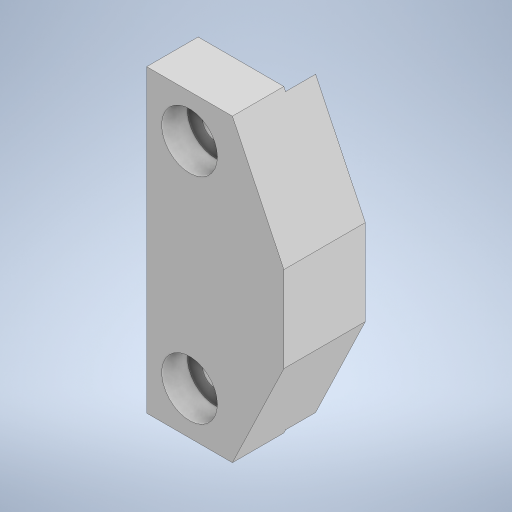
# Autodesk Inventor part: Clamp
Saved by Autodesk Inventor 2024 (Build 280153000, 153)
## iProperties
Created: 2024-09-24
Part Number: Clamp
Material: Generic
Document SubType Name: Modeling
Designer: Kemper Room 121
Density: 1 g/cm^3
Appearance: Default
Author: Kemper Room 121
Autodesk Inventor part; units mm, degrees
ref_plane "YZ Plane" through (0, 0, 0) normal (1, 0, 0) x (0, 1, 0)
ref_plane "XZ Plane" through (0, 0, 0) normal (0, 1, 0) x (-1, 0, 0)
ref_plane "XY Plane" through (0, 0, 0) normal (0, 0, 1) x (1, 0, 0)
sketch "Sketch1" plane through (0, 0, 0) normal (0, 0, 1) x (1, 0, 0)
  line L0 (0, 0) -> (0, 5)
  line L1 (0, 5) -> (0, 30)
  line L2 (0, 30) -> (0, 35)
  line L3 (0, 35) -> (10, 35)
  line L4 (10, 35) -> (10, 0)
  line L5 (10, 0) -> (0, 0)
  line L6 (0, 35) -> (5, 35)
  line L7 (5, 35) -> (5, 0)
  circle A0 centre (5, 30) radius 1.5
  circle A1 centre (5, 5) radius 1.5
  line L8 (5, 17.5) -> (10, 17.5)
  line L9 (10, 17.5) -> (16, 17.5)
  line L10 (16, 17.5) -> (16, 12.5)
  line L11 (16, 17.5) -> (16, 22.5)
  line L12 (16, 22.5) -> (10, 35)
  line L13 (16, 12.5) -> (10, 0)
  dimension "d0" = 5
  dimension "d1" = 25
  dimension "d2" = 5
  dimension "d3" = 10
  dimension "d4" = 5
  dimension "d5" = 3
  dimension "d6" = 3
  dimension "d7" = 6
  dimension "d8" = 5
  dimension "d9" = 5
  constraints: 28 end point, 4 midpoint, 4 point on line, 3 perpendicular, 3 vertical, 2 centre point, 1 horizontal
  measures "d0" distance of L0.start L0.end
  measures "d1" distance of L0.end L1.end
  measures "d2" distance of L1.end L2.end
  measures "d3" distance of L2.end L3.end
  measures "d4" distance of L2.end L6.end
  measures "d5" diameter of A0
  measures "d6" diameter of A1
  measures "d7" distance of L8.end L9.end
  measures "d8" distance of L9.end L10.end
  measures "d9" distance of L9.end L11.end
extrude "Extrusion1" add sketch "Sketch1" along normal blind 6 contours L0 L1 L2 L3 L7 A0 A1 L5 | L7 A1 L8 L4 L5 | L4 L9 L10 L13 | L8 L7 A0 L3 L4 | L4 L12 L11 L9
sketch "Sketch2" plane through (0, 0, 0) normal (0, 0, -1) x (-1, 0, 0)
  line L0 (0, 35) -> (0, 0) projected
  line L1 (-10, 35) -> (0, 35) projected
  line L2 (-16, 22.5) -> (-10, 35) projected
  line L3 (-16, 12.5) -> (-16, 22.5) projected
  line L4 (-10, 0) -> (-16, 12.5) projected
  line L5 (0, 0) -> (-10, 0) projected
  circle A0 centre (-5, 30) radius 1.5 projected
  circle A1 centre (-5, 5) radius 1.5 projected
  line L6 (-10, 0) -> (-16, 12.5) projected
  line L7 (-10, 35) -> (-10, 0)
  line L8 (-10, 0) -> (-16, 12.5)
  line L9 (-16, 12.5) -> (-16, 22.5)
  line L10 (-10, 35) -> (-16, 22.5)
  line L11 (-10.2, 34.5833) -> (-10.2, 0.4167)
  point P0 (-10.2, 0.4167)
  dimension "d54" = 0.2
  constraints: 10 end point, 2 parallel, 2 point on line, 1 collinear, 1 vertical
  measures "d54" distance between parallel lines of L7 L11
extrude "Extrusion2" add sketch "Sketch2" along normal blind 3.5 contours L11 L4 L3 L2
sketch "Sketch3" plane through (0, 0, 6) normal (0, 0, 1) x (1, 0, 0)
  line L0 (0, 35) -> (0, 0) projected
  line L1 (0, 0) -> (10, 0) projected
  line L2 (10, 0) -> (16, 12.5) projected
  line L3 (16, 12.5) -> (16, 22.5) projected
  line L4 (16, 22.5) -> (10, 35) projected
  line L5 (10, 35) -> (0, 35) projected
  circle A0 centre (5, 30) radius 1.5 projected
  circle A1 centre (5, 5) radius 1.5 projected
  circle A2 centre (5, 30) radius 3.25
  circle A3 centre (5, 5) radius 3.25
  dimension "d14" = 6.5
  dimension "d17" = 6.5
  constraints: 2 centre point, 2 coincident
  measures "d14" diameter of A2
  measures "d17" diameter of A3
extrude "Extrusion3" cut sketch "Sketch3" against normal blind 3 contours A0 | A2 | A3
sketch "Sketch4" plane through (0, 0, -3.5) normal (0, 0, -1) x (-1, 0, 0)
  line L0 (-10.2, 34.5833) -> (-16, 22.5) projected
  line L1 (-16, 22.5) -> (-16, 12.5) projected
  line L2 (-16, 12.5) -> (-10.2, 0.4167) projected
  line L3 (0, 0) -> (-10, 0) projected
  line L4 (0, 35) -> (0, 0) projected
  line L5 (-10, 35) -> (0, 35) projected
  circle A0 centre (-5, 30) radius 1.5 projected
  circle A1 centre (-5, 5) radius 1.5 projected
  line L6 (-15.8046, 22.9071) -> (-13.1, 21.609)
  line L7 (-15.8046, 12.0929) -> (-13.1, 13.391)
  circle A2 centre (-13.1, 13.391) radius 1
  circle A3 centre (-13.1, 21.609) radius 1
  line L8 (-10.2, 34.5833) -> (-10.2, 0.4167) projected
  line L9 (-10, 0) -> (-10.2, 0.4167) projected
  line L10 (-10.2, 34.5833) -> (-10, 35) projected
  line L11 (-10.2, 0.4167) -> (-10.2, 34.5833) projected
  dimension "d39" = 3
  dimension "d41" = 90
  dimension "d42" = 3
  dimension "d43" = 90
  dimension "d45" = 2.9
  dimension "d46" = 2
  dimension "d47" = 2
  dimension "d52" = 8.2179
  dimension "d55" = 2.9
  dimension "d56" = 0.2
  dimension "d57" = 6
  constraints: 4 end point, 2 centre point, 2 coincident, 2 point on line
  measures "d39" distance of L6.start L6.end
  measures "d41" angle of L0 L6
  measures "d42" distance of L7.start L7.end
  measures "d43" angle of L2 L7
  measures "d45" distance from line of L1 L7.end
  measures "d46" diameter of A2
  measures "d47" diameter of A3
  measures "d52" distance of L6.end L7.end
  measures "d55" distance from line of L1 L6.end
  measures "d56" horizontal distance of L5.start L8.start
  measures "d57" horizontal distance of L0.end L5.start
extrude "Extrusion4" cut sketch "Sketch4" against normal blind 8 contours A3 | A2
equation "\"d2\" = d0"
equation "\"d4\" = 0.5 * d3"
equation "\"d9\" = d8"
equation "\"d39\" = 0.5 * d36"
equation "\"d42\" = d39"
equation "\"d45\" = d55"
equation "\"d55\" = -0.5 * d56 + 0.5 * d57"
equation "\"d36\" = 6"
body "Solid1"
